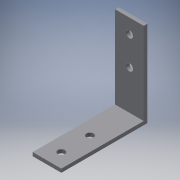
# Autodesk Inventor part: 15102898-16-P-0510
Saved by Autodesk Inventor 2017 (Build 210142000, 142)
## iProperties
Created: 2016-10-08
Part Number: 15102898-16-P-0510
Material: Stainless Steel
Document SubType Name: Modeling
Designer: 15102898
Density: 8 g/cm^3
Appearance: Semi-Polished
Author: 15102898
Autodesk Inventor part; units mm, degrees
ref_plane "YZ Plane" through (0, 0, 0) normal (1, 0, 0) x (0, 1, 0)
ref_plane "XZ Plane" through (0, 0, 0) normal (0, 1, 0) x (-1, 0, 0)
ref_plane "XY Plane" through (0, 0, 0) normal (0, 0, 1) x (1, 0, 0)
sketch "Sketch1" plane through (0, 0, 0) normal (0, 0, 1) x (1, 0, 0)
  line L0 (0, 0) -> (25.4, 0)
  line L1 (25.4, 0) -> (25.4, -76.2)
  line L2 (25.4, -76.2) -> (0, -76.2)
  line L3 (0, -76.2) -> (0, 0)
  circle A0 centre (12.7, -12.7) radius 3.175
  circle A1 centre (12.7, -38.1) radius 3.175
  dimension "d0" = 25.4
  dimension "d1" = 76.2
  dimension "d2" = 6.35
  dimension "d3" = 6.35
  dimension "d4" = 12.7
  dimension "d5" = 12.7
  dimension "d6" = 12.7
  dimension "d7" = 25.4
  constraints: 8 end point, 2 centre point, 2 parallel, 1 horizontal, 1 perpendicular
  measures "d0" distance of L1.end L2.end
  measures "d1" distance of L0.end L1.end
  measures "d2" diameter of A0
  measures "d3" diameter of A1
  measures "d4" distance from line of L1 A0.centre
  measures "d5" distance from line of L0 A0.centre
  measures "d6" distance from line of L1 A1.centre
  measures "d7" distance of A0.centre A1.centre
extrude "Extrusion1" add sketch "Sketch1" along normal blind 3.175
sketch "Sketch2" plane through (0, 0, 3.175) normal (0, 0, 1) x (1, 0, 0)
  line L0 (25.4, -76.2) -> (25.4, 0) projected
  line L1 (0, 0) -> (0, -76.2) projected
  line L2 (25.4, -76.2) -> (0, -76.2)
  line L3 (0, -76.2) -> (0, -73.025)
  line L4 (0, -73.025) -> (25.4, -73.025)
  line L5 (25.4, -73.025) -> (25.4, -76.2)
  dimension "d10" = 3.175
  constraints: 8 end point, 2 parallel, 1 horizontal, 1 perpendicular, 1 point on line
  measures "d10" distance of L2.end L3.end
extrude "Extrusion2" add sketch "Sketch2" along normal blind 73.025
sketch "Sketch3" plane through (0, -73.025, 3.175) normal (0, 1, 0) x (1, 0, 0)
  circle A0 centre (12.7, -60.325) radius 3.175
  circle A1 centre (12.7, -34.925) radius 3.175
  line L0 (0, 0) -> (0, -73.025) projected
  line L1 (25.4, -73.025) -> (0, -73.025) projected
  point P0 (0, 3.175)
  dimension "d13" = 6.35
  dimension "d14" = 6.35
  dimension "d15" = 12.7
  dimension "d16" = 12.7
  dimension "d17" = 12.7
  dimension "d18" = 25.4
  constraints: 2 centre point
  measures "d13" diameter of A1
  measures "d14" diameter of A0
  measures "d15" distance from line of L0 A0.centre
  measures "d16" distance from line of L1 A0.centre
  measures "d17" distance from line of L0 A1.centre
  measures "d18" distance of A0.centre A1.centre
extrude "Extrusion3" cut sketch "Sketch3" against normal blind 73.025
body "Solid1"
